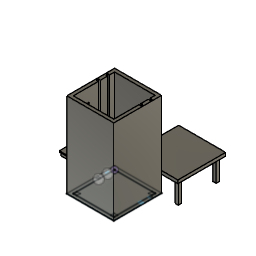
Card reader (Autodesk Fusion 360 design; units mm, degrees)
Autodesk Fusion 360 part; units mm, degrees
sketch "Sketch1" plane through (0, 0, 0) normal (0, 0, 1) x (1, 0, 0)
  line L0 (0, 0) -> (37.25, 0)
  line L1 (37.25, 0) -> (37.25, -38)
  line L2 (37.25, -38) -> (0, -38)
  line L3 (0, -38) -> (0, 0)
  line L4 (37.25, -14.85) -> (37.25, -13)
  line L5 (-3, 3) -> (40.25, 3)
  line L6 (40.25, 3) -> (40.25, -41)
  line L7 (40.25, -41) -> (-3, -41)
  line L8 (-3, -41) -> (-3, 3)
  line L9 (37.25, -14.85) -> (39.25, -14.85)
  line L10 (39.25, -14.85) -> (39.25, -13)
  line L11 (39.25, -13) -> (37.25, -13)
  line L12 (37.25, -13) -> (37.25, -14.85)
  line L13 (0, -14.85) -> (-2, -14.85)
  line L14 (-2, -14.85) -> (-2, -13)
  line L15 (-2, -13) -> (0, -13)
  line L16 (0, -13) -> (0, -14.85)
  line L17 (0, -4.5) -> (-1.75, -4.5)
  line L18 (-1.75, -4.5) -> (-1.75, -6.35)
  line L19 (-1.75, -6.35) -> (0, -6.35)
  line L20 (37.25, -6.35) -> (39, -6.35)
  line L21 (39, -6.35) -> (39, -4.5)
  line L22 (39, -4.5) -> (37.25, -4.5)
  line L23 (37.25, -4.5) -> (37.25, -6.35)
  line L24 (0.09, -0.09) -> (37.52, -0.09)
  line L25 (37.52, -0.09) -> (37.52, -37.91)
  line L26 (37.52, -37.91) -> (0.09, -37.91)
  line L27 (0.09, -37.91) -> (0.09, -0.09)
  line L28 (0.09, -14.75) -> (0.09, -13.1)
  line L29 (37.52, -0.09) -> (34.52, -0.09)
  line L30 (34.52, -0.09) -> (34.52, -3.09)
  line L31 (34.52, -3.09) -> (37.52, -3.09)
  line L32 (37.52, -3.09) -> (37.52, -0.09)
  line L33 (0.09, -0.09) -> (3.09, -0.09)
  line L34 (3.09, -0.09) -> (3.09, -3.09)
  line L35 (3.09, -3.09) -> (0.09, -3.09)
  line L36 (0.09, -3.09) -> (0.09, -0.09)
  line L37 (0.09, -37.91) -> (3.09, -37.91)
  line L38 (3.09, -37.91) -> (3.09, -34.91)
  line L39 (3.09, -34.91) -> (0.09, -34.91)
  line L40 (0.09, -34.91) -> (0.09, -37.91)
  line L41 (37.52, -37.91) -> (34.52, -37.91)
  line L42 (34.52, -37.91) -> (34.52, -34.91)
  line L43 (34.52, -34.91) -> (37.52, -34.91)
  line L44 (37.52, -34.91) -> (37.52, -37.91)
  dimension "d1" = 37.25
  dimension "d2" = 38
  dimension "d9" = 43.25
  dimension "d10" = 44
  dimension "d11" = 3
  dimension "d12" = 3
  dimension "d17" = 2
  dimension "d19" = 2
  dimension "d20" = 1.85
  dimension "d21" = 13
  dimension "d28" = 1.75
  dimension "d29" = 1.85
  dimension "d30" = 1.75
  dimension "d31" = 1.85
  dimension "d32" = 4.5
  dimension "d33" = 13
  dimension "d34" = 1.85
  dimension "d46" = 37.43
  dimension "d47" = 37.82
  dimension "d52" = 0.09
  dimension "d53" = 0.09
  dimension "d58" = 4.5
  dimension "d86" = 3
  dimension "d87" = 3
  dimension "d88" = 3
  dimension "d89" = 3
  dimension "d90" = 3
  dimension "d91" = 3
  dimension "d92" = 3
  dimension "d93" = 3
  constraint horizontal L0
  constraint vertical L1
  constraint horizontal L2
  constraint vertical L3
  constraint coincident L0.start L3.end
  constraint coincident L1 L4.end
  constraint horizontal L5
  constraint vertical L6
  constraint horizontal L7
  constraint vertical L8
  constraint horizontal L9
  constraint vertical L10
  constraint horizontal L11
  constraint horizontal L13
  constraint vertical L14
  constraint horizontal L15
  constraint vertical L16
  constraint coincident L3 L13.start
  constraint vertical L18
  constraint horizontal L19
  constraint coincident L3 L17.start
  constraint horizontal L20
  constraint vertical L21
  constraint horizontal L22
  constraint coincident L1 L20.start
  constraint horizontal L24
  constraint vertical L25
  constraint horizontal L26
  constraint vertical L27
  constraint vertical L28
  constraint coincident L27 L28.end
  constraint horizontal L29
  constraint vertical L30
  constraint horizontal L31
  constraint vertical L32
  constraint horizontal L33
  constraint vertical L34
  constraint horizontal L35
  constraint vertical L36
  constraint horizontal L37
  constraint vertical L38
  constraint horizontal L39
  constraint vertical L40
  constraint horizontal L41
  constraint vertical L42
  constraint horizontal L43
  constraint vertical L44
  measures "d1" distance of L0.start L0.end
  measures "d2" distance of L0.start L2.end
  measures "d9" distance of L5.start L5.end
  measures "d10" distance of L5.start L7.end
  measures "d11" distance of L0 L5
  measures "d12" distance of L3 L8
  measures "d17" distance of L4.start L9.end
  measures "d19" distance of L13.start L13.end
  measures "d20" distance of L13.start L15.end
  measures "d21" distance of L0.start L15.end
  measures "d28" distance of L17.start L17.end
  measures "d29" distance of L17.start L19.end
  measures "d30" distance of L20.start L20.end
  measures "d31" distance of L20.start L22.end
  measures "d32" distance of L0.start L17.start
  measures "d33" distance of L0.end L4.end
  measures "d34" distance of L9.end L10.end
  measures "d46" distance of L24.start L24.end
  measures "d47" distance of L24.start L26.end
  measures "d52" distance of L3 L27
  measures "d53" distance of L0 L24
  measures "d58" distance of L0 L22
  measures "d86" distance of L24.end L29.end
  measures "d87" distance of L24.end L31.end
  measures "d88" distance of L24.start L33.end
  measures "d89" distance of L24.start L35.end
  measures "d90" distance of L26.end L37.end
  measures "d91" distance of L26.end L39.end
  measures "d92" distance of L25.end L41.end
  measures "d93" distance of L25.end L43.end
extrude "Extrude1" add sketch "Sketch1" along normal blind 2 contours L0 L1 L2 L3 L16 L24 L26 L27 L28 L29 L33 L36 L37 L40 L41 | L3 L17 L18 L19 | L1 L24 L25 L29 L31 L32 | L1 L24 L29 L30 L31 | L1 L22 L25 L31 | L1 L4 L12 L23 L24 L26 L27 L28 L30 L31 L34 L35 L38 L39 L42 L43 | L3 L13 L14 L15 L16 | L1 L20 L22 L23 L25 | L24 L27 L33 L34 L35 L36 | L1 L11 L20 L25 | L20 L21 L22 L25 | L1 L4 L9 L11 L12 L25 | L1 L9 L25 L43 | L9 L10 L11 L25 | L1 L26 L41 L42 L43 | L1 L25 L26 L41 L43 L44 | L26 L27 L37 L38 L39 L40 | L5 L6 L7 L8 makes body 1
extrude "Extrude2" add sketch "Sketch1" along normal blind 78 contours L1 L24 L25 L29 L31 L32 | L1 L22 L25 L31 | L1 L11 L20 L25 | L1 L9 L25 L43 | L1 L25 L26 L41 L43 L44 | L5 L6 L7 L8 bodies 1
sketch "Sketch3" plane through (-3, 0, 0) normal (-1, 0, 0) x (0, -1, 0)
  line L0 (-3, 0) -> (41, 0)
  line L1 (41, 0) -> (41, 78)
  line L2 (41, 78) -> (-3, 78)
  line L3 (-3, 78) -> (-3, 0)
  line L4 (23.5, 26.5) -> (33, 26.5)
  line L5 (33, 26.5) -> (33, 38.5)
  line L6 (33, 38.5) -> (23.5, 38.5)
  line L7 (23.5, 38.5) -> (23.5, 26.5)
  line L8 (41, 0) -> (-3, 0)
  line L9 (23.5, 53.5) -> (33, 53.5)
  line L10 (33, 53.5) -> (33, 65.5)
  line L11 (33, 65.5) -> (23.5, 65.5)
  line L12 (23.5, 65.5) -> (23.5, 53.5)
  dimension "d36" = 38.5
  dimension "d37" = 12
  dimension "d38" = 9.5
  dimension "d39" = 36
  dimension "d40" = 9.5
  dimension "d41" = 12
  dimension "d42" = 36
  dimension "d43" = 65.5
  constraint horizontal L4
  constraint vertical L5
  constraint horizontal L6
  constraint vertical L7
  constraint horizontal L9
  constraint vertical L10
  constraint horizontal L11
  constraint vertical L12
  measures "d36" distance of L6 L8
  measures "d37" distance of L4.start L6.end
  measures "d38" distance of L4.start L4.end
  measures "d39" distance of L3 L5
  measures "d40" distance of L9.start L9.end
  measures "d41" distance of L9.start L11.end
  measures "d42" distance of L3 L10
  measures "d43" distance of L8 L11
extrude "Extrude3" cut sketch "Sketch3" against normal blind 3 contours L4 L5 L6 L7 | L9 L10 L11 L12 bodies 1
extrude "Extrude4" add sketch "Sketch1" against normal blind 0.5 separate body contours L1 L24 L25 L29 L31 L32 | L1 L24 L29 L30 L31 | L1 L22 L25 L31 | L1 L4 L12 L23 L24 L26 L27 L28 L30 L31 L34 L35 L38 L39 L42 L43 | L1 L20 L22 L23 L25 | L24 L27 L33 L34 L35 L36 | L1 L11 L20 L25 | L1 L4 L9 L11 L12 L25 | L1 L9 L25 L43 | L1 L26 L41 L42 L43 | L1 L25 L26 L41 L43 L44 | L26 L27 L37 L38 L39 L40 makes body 2
extrude "Extrude8" add sketch "Sketch1" against normal blind 20 separate body contours L1 L24 L25 L29 L31 L32 | L1 L24 L29 L30 L31 | L24 L27 L33 L34 L35 L36 | L1 L26 L41 L42 L43 | L1 L25 L26 L41 L43 L44 | L26 L27 L37 L38 L39 L40 makes body 3 at (37.52, -35.91, -13.3333) makes body 4 at (0.09, -2.09, -6.6667) makes body 5 at (35.52, -0.09, -13.3333) makes body 6 at (0.09, -36.91, -6.6667)
combine "Combine1" operation add target body 2 tool bodies 4 5 3 6
move_body "Move1" bodies 2 to x (1, 0, 0) y (0, 1, 0) z (0, 0, 1) at (0, 59, 0)
sketch "Sketch4" plane through (0, 0, 0) normal (0, 0, 1) x (-1, 0, 0)
  line L0 (-0.09, -21.09) -> (-37.52, -21.09)
  line L1 (-37.52, -21.09) -> (-37.52, -58.91)
  line L2 (-37.52, -58.91) -> (-0.09, -58.91)
  line L3 (-0.09, -58.91) -> (-0.09, -21.09)
  line L4 (-40.25, -17.99) -> (3, -17.99)
  line L5 (3, -17.99) -> (3, -61.99)
  line L6 (3, -61.99) -> (-40.25, -61.99)
  line L7 (-40.25, -61.99) -> (-40.25, -17.99)
  dimension "d67" = 43.25
  dimension "d68" = 44
  dimension "d72" = 3.1
  dimension "d73" = 3.08
  constraint horizontal L4
  constraint vertical L5
  constraint horizontal L6
  constraint vertical L7
  measures "d67" distance of L4.start L4.end
  measures "d68" distance of L4.start L6.end
  measures "d72" distance of L0 L4
  measures "d73" distance of L2 L6
extrude "Extrude5" add sketch "Sketch4" along normal blind 3 contours L0 L1 L2 L3 | L4 L5 L6 L7 bodies 2
sketch "Sketch5" plane through (0, 0, 0) normal (0, 0, 1) x (1, 0, 0)
  line L0 (-26.8002, -13.5841) -> (-35.9002, -13.5841)
  line L1 (-35.9002, -13.5841) -> (-35.9002, -1.9841)
  line L2 (-35.9002, -1.9841) -> (-26.8002, -1.9841)
  line L3 (-26.8002, -1.9841) -> (-26.8002, -13.5841)
  dimension "d76" = 9.1
  dimension "d77" = 11.6
  constraint horizontal L0
  constraint vertical L1
  constraint horizontal L2
  constraint vertical L3
  measures "d76" distance of L0.start L0.end
  measures "d77" distance of L0.start L2.end
extrude "Extrude6" add sketch "Sketch5" along normal blind 3 separate body makes body 7
sketch "Sketch6" plane through (0, 0, 3) normal (0, 0, 1) x (-1, 0, 0)
  line L0 (26.8002, 1.9841) -> (35.9002, 1.9841)
  line L1 (35.9002, 1.9841) -> (35.9002, 13.5841)
  line L2 (35.9002, 13.5841) -> (26.8002, 13.5841)
  line L3 (26.8002, 13.5841) -> (26.8002, 1.9841)
  line L4 (26.1002, 14.2841) -> (36.6002, 14.2841)
  line L5 (36.6002, 14.2841) -> (36.6002, 1.2841)
  line L6 (36.6002, 1.2841) -> (26.1002, 1.2841)
  line L7 (26.1002, 1.2841) -> (26.1002, 14.2841)
  dimension "d80" = 10.5
  dimension "d81" = 13
  dimension "d82" = 0.7
  dimension "d83" = 0.7
  constraint horizontal L4
  constraint vertical L5
  constraint horizontal L6
  constraint vertical L7
  measures "d80" distance of L4.start L4.end
  measures "d81" distance of L4.start L6.end
  measures "d82" distance of L2 L4
  measures "d83" distance of L3 L7
extrude "Extrude7" add sketch "Sketch6" 1 faces at (-29.8335, -9.7175, 3) along normal blind 1 contours L0 L1 L2 L3 | L4 L5 L6 L7 on bodies 7 bodies 7
equation "d1 = 41.25 mm - d19 * 2"
equation "d2 = 25 mm + d21"
equation "d9 = d1 + d11 * 2"
equation "d10 = d2 + d11 * 2"
equation "d12 = d11"
equation "d17 = d19"
equation "d20 = d29"
equation "d28 = d19 - 0.25 mm"
equation "d30 = d28"
equation "d31 = d29"
equation "d33 = d21"
equation "d34 = d20"
equation "d40 = d38"
equation "d41 = d37"
equation "d46 = d1 - -2 * d52"
equation "d47 = d2 - 2 * d52"
equation "d51 = d32"
equation "d53 = d52"
equation "d56 = d51"
equation "d58 = d56"
